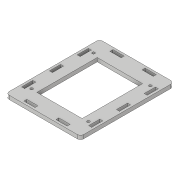
# Autodesk Inventor part: tapa1
Saved by Autodesk Inventor 2019 (Build 230136000, 136)
## iProperties
Created: 2018-09-17
Part Number: tapa1
Material: Genérico
Document SubType Name: Modeling
Designer: lmacia
Density: 1 g/cm^3
Appearance: Valor por defecto
Author: lmacia
Autodesk Inventor part; units mm, degrees
ref_plane "YZ Plane" through (0, 0, 0) normal (1, 0, 0) x (0, 1, 0)
ref_plane "XZ Plane" through (0, 0, 0) normal (0, 1, 0) x (-1, 0, 0)
ref_plane "XY Plane" through (0, 0, 0) normal (0, 0, 1) x (1, 0, 0)
sketch "Boceto1" plane through (0, 0, 0) normal (0, 1, 0) x (-1, 0, 0)
  line L0 (25.8375, 17.5875) -> (25.7625, 17.5875)
  line L1 (25.7625, 17.5875) -> (25.7625, 26.5875)
  line L2 (25.7625, 26.5875) -> (25.8375, 26.5875)
  line L3 (25.7625, 26.5875) -> (28.0125, 26.5875)
  line L4 (28.0875, 26.5875) -> (28.1625, 26.5875)
  line L5 (28.1625, 17.5875) -> (28.0875, 17.5875)
  line L6 (28.0125, 17.5875) -> (25.7625, 17.5875)
  line L7 (25.8148, -4.7625) -> (25.7398, -4.7625)
  line L8 (25.7398, -4.7625) -> (25.7398, 4.2375)
  line L9 (25.7398, 4.2375) -> (25.8148, 4.2375)
  line L10 (25.7398, 4.2375) -> (28.1625, 4.2375)
  line L11 (28.1625, -4.7625) -> (28.0875, -4.7625)
  line L12 (28.0875, -4.7625) -> (25.8148, -4.7625)
  line L13 (23.8875, 23.8875) -> (23.8517, 23.6157)
  line L14 (23.8517, 23.6157) -> (23.7468, 23.3625)
  line L15 (23.754, 23.357) -> (23.5871, 23.1396)
  line L16 (23.58, 23.145) -> (23.3625, 22.9782)
  line L17 (23.3625, 22.9782) -> (23.1093, 22.8733)
  line L18 (23.1093, 22.8733) -> (22.8375, 22.8375)
  line L19 (22.8375, 22.8375) -> (22.5657, 22.8733)
  line L20 (22.5657, 22.8733) -> (22.3125, 22.9782)
  line L21 (22.3125, 22.9782) -> (22.095, 23.145)
  line L22 (22.0879, 23.1396) -> (21.921, 23.357)
  line L23 (21.9282, 23.3625) -> (21.8233, 23.6157)
  line L24 (21.8233, 23.6157) -> (21.7875, 23.8875)
  line L25 (21.7875, 23.8875) -> (21.8233, 24.1593)
  line L26 (21.8233, 24.1593) -> (21.9282, 24.4125)
  line L27 (21.9282, 24.4125) -> (22.095, 24.63)
  line L28 (22.095, 24.63) -> (22.3125, 24.7968)
  line L29 (22.3125, 24.7968) -> (22.5657, 24.9017)
  line L30 (22.5657, 24.9017) -> (22.8375, 24.9375)
  line L31 (22.8387, 24.9464) -> (23.1104, 24.9106)
  line L32 (23.1093, 24.9017) -> (23.3625, 24.7968)
  line L33 (23.3625, 24.7968) -> (23.58, 24.63)
  line L34 (23.58, 24.63) -> (23.7468, 24.4125)
  line L35 (23.7468, 24.4125) -> (23.8517, 24.1593)
  line L36 (23.8517, 24.1593) -> (23.8875, 23.8875)
  line L37 (18.225, 24.3) -> (18.225, -24.3)
  line L38 (18.225, -24.3) -> (-18.225, -24.3)
  line L39 (-18.225, -24.3) -> (-18.225, 24.3)
  line L40 (-18.225, 24.3) -> (18.225, 24.3)
  line L41 (-25.8375, 26.5875) -> (-25.7625, 26.5875)
  line L42 (-25.7625, 26.5875) -> (-25.7625, 17.5875)
  line L43 (-25.7625, 17.5875) -> (-25.8375, 17.5875)
  line L44 (-25.8375, 17.5875) -> (-28.0875, 17.5875)
  line L45 (-28.0875, 17.5875) -> (-28.1625, 17.5875)
  line L46 (-28.1625, 17.5875) -> (-28.1625, 26.5875)
  line L47 (-28.1625, 26.5875) -> (-28.0875, 26.5875)
  line L48 (-28.0875, 26.5875) -> (-25.8375, 26.5875)
  line L49 (-25.8375, -27.1125) -> (-28.0875, -27.1125)
  line L50 (-28.0875, -27.1125) -> (-28.1625, -27.1125)
  line L51 (-28.1625, -27.1125) -> (-28.1625, -18.1125)
  line L52 (-28.1625, -18.1125) -> (-28.0875, -18.1125)
  line L53 (-28.0875, -18.1125) -> (-25.8375, -18.1125)
  line L54 (-25.8375, -18.1125) -> (-25.7625, -18.1125)
  line L55 (-25.7625, -18.1125) -> (-25.7625, -27.1125)
  line L56 (-25.7625, -27.1125) -> (-25.8375, -27.1125)
  line L57 (-22.5657, 22.8733) -> (-22.8375, 22.8375)
  line L58 (-22.8375, 22.8375) -> (-23.1093, 22.8733)
  line L59 (-23.1093, 22.8733) -> (-23.3625, 22.9782)
  line L60 (-23.3625, 22.9782) -> (-23.58, 23.145)
  line L61 (-23.58, 23.145) -> (-23.7468, 23.3625)
  line L62 (-23.7551, 23.3591) -> (-23.86, 23.6123)
  line L63 (-23.8517, 23.6157) -> (-23.8875, 23.8875)
  line L64 (-23.8875, 23.8875) -> (-23.8517, 24.1593)
  line L65 (-23.8517, 24.1593) -> (-23.7468, 24.4125)
  line L66 (-23.7468, 24.4125) -> (-23.58, 24.63)
  line L67 (-23.58, 24.63) -> (-23.3625, 24.7968)
  line L68 (-23.3625, 24.7968) -> (-23.1093, 24.9017)
  line L69 (-23.1093, 24.9017) -> (-22.8375, 24.9375)
  line L70 (-22.8363, 24.9464) -> (-22.5646, 24.9106)
  line L71 (-22.5657, 24.9017) -> (-22.3125, 24.7968)
  line L72 (-22.3125, 24.7968) -> (-22.095, 24.63)
  line L73 (-22.095, 24.63) -> (-21.9282, 24.4125)
  line L74 (-21.9282, 24.4125) -> (-21.8233, 24.1593)
  line L75 (-21.8233, 24.1593) -> (-21.7875, 23.8875)
  line L76 (-21.7875, 23.8875) -> (-21.8233, 23.6157)
  line L77 (-21.8233, 23.6157) -> (-21.9282, 23.3625)
  line L78 (-21.9282, 23.3625) -> (-22.095, 23.145)
  line L79 (-22.095, 23.145) -> (-22.3125, 22.9782)
  line L80 (-22.3091, 22.9699) -> (-22.5623, 22.865)
  line L81 (-28.1625, -4.7625) -> (-28.1625, 4.2375)
  line L82 (-28.1625, 4.2375) -> (-28.0875, 4.2375)
  line L83 (-28.0875, 4.2375) -> (-25.8375, 4.2375)
  line L84 (-25.8375, 4.2375) -> (-25.7625, 4.2375)
  line L85 (-25.7625, 4.2375) -> (-25.7625, -4.7625)
  line L86 (-25.7625, -4.7625) -> (-25.8375, -4.7625)
  line L87 (-25.8375, -4.7625) -> (-28.0875, -4.7625)
  line L88 (-28.0875, -4.7625) -> (-28.1625, -4.7625)
  line L89 (-22.5657, -27.0017) -> (-22.8375, -27.0375)
  line L90 (-22.8375, -27.0375) -> (-23.1093, -27.0017)
  line L91 (-23.1093, -27.0017) -> (-23.3625, -26.8968)
  line L92 (-23.3625, -26.8968) -> (-23.58, -26.73)
  line L93 (-23.58, -26.73) -> (-23.7468, -26.5125)
  line L94 (-23.7551, -26.5159) -> (-23.86, -26.2627)
  line L95 (-23.8517, -26.2593) -> (-23.8875, -25.9875)
  line L96 (-23.8875, -25.9875) -> (-23.8517, -25.7157)
  line L97 (-23.8517, -25.7157) -> (-23.7468, -25.4625)
  line L98 (-23.7468, -25.4625) -> (-23.58, -25.245)
  line L99 (-23.58, -25.245) -> (-23.3625, -25.0782)
  line L100 (-23.3625, -25.0782) -> (-23.1093, -24.9733)
  line L101 (-23.1093, -24.9733) -> (-22.8375, -24.9375)
  line L102 (-22.8363, -24.9286) -> (-22.5646, -24.9644)
  line L103 (-22.5657, -24.9733) -> (-22.3125, -25.0782)
  line L104 (-22.3125, -25.0782) -> (-22.095, -25.245)
  line L105 (-22.095, -25.245) -> (-21.9282, -25.4625)
  line L106 (-21.9282, -25.4625) -> (-21.8233, -25.7157)
  line L107 (-21.8233, -25.7157) -> (-21.7875, -25.9875)
  line L108 (-21.7875, -25.9875) -> (-21.8233, -26.2593)
  line L109 (-21.8233, -26.2593) -> (-21.9282, -26.5125)
  line L110 (-21.9282, -26.5125) -> (-22.095, -26.73)
  line L111 (-22.0896, -26.7371) -> (-22.307, -26.904)
  line L112 (-22.3125, -26.8968) -> (-22.5657, -27.0017)
  line L113 (8.4187, -36.0375) -> (8.4187, -33.7875)
  line L114 (8.4187, -33.7875) -> (8.4187, -33.7125)
  line L115 (8.4187, -33.7125) -> (17.4187, -33.7125)
  line L116 (17.4187, -33.7125) -> (17.4187, -33.7875)
  line L117 (17.4187, -33.7875) -> (17.4187, -36.0375)
  line L118 (17.4187, -36.0375) -> (17.4187, -36.1125)
  line L119 (17.4187, -36.1125) -> (8.4187, -36.1125)
  line L120 (8.4187, -36.1125) -> (8.4187, -36.0375)
  line L121 (8.4187, 33.1875) -> (8.4187, 33.2625)
  line L122 (8.4187, 33.1875) -> (8.4187, 35.5125)
  line L123 (8.4187, 35.5125) -> (8.4187, 35.5875)
  line L124 (17.4187, 35.5875) -> (17.4187, 35.5125)
  line L125 (17.4187, 33.1875) -> (8.4187, 33.1875)
  line L126 (-17.4188, 33.1875) -> (-17.4188, 33.2625)
  line L127 (-17.4188, 33.2625) -> (-17.4188, 35.5125)
  line L128 (-17.4188, 35.5125) -> (-17.4188, 35.5875)
  line L129 (-17.4188, 35.5875) -> (-8.4188, 35.5875)
  line L130 (-8.4188, 35.5875) -> (-8.4188, 35.5125)
  line L131 (-8.4188, 35.5125) -> (-8.4188, 33.2625)
  line L132 (-8.4188, 33.2625) -> (-8.4188, 33.1875)
  line L133 (-8.4188, 33.1875) -> (-17.4188, 33.1875)
  line L134 (-8.4188, -33.7125) -> (-8.4188, -33.7875)
  line L135 (-8.4188, -33.7875) -> (-8.4188, -36.0375)
  line L136 (-8.4188, -36.0375) -> (-8.4188, -36.1125)
  line L137 (-8.4188, -36.1125) -> (-17.4188, -36.1125)
  line L138 (-17.4188, -36.1125) -> (-17.4188, -36.0375)
  line L139 (-17.4188, -36.0375) -> (-17.4188, -33.7875)
  line L140 (-17.4188, -33.7875) -> (-17.4188, -33.7125)
  line L141 (-17.4188, -33.7125) -> (-8.4188, -33.7125)
  line L142 (23.8517, -25.7157) -> (23.8875, -25.9875)
  line L143 (23.8875, -25.9875) -> (23.8517, -26.2593)
  line L144 (23.8517, -26.2593) -> (23.7468, -26.5125)
  line L145 (23.7468, -26.5125) -> (23.58, -26.73)
  line L146 (23.5854, -26.7371) -> (23.368, -26.904)
  line L147 (23.3625, -26.8968) -> (23.1093, -27.0017)
  line L148 (23.1093, -27.0017) -> (22.8375, -27.0375)
  line L149 (22.8375, -27.0375) -> (22.5657, -27.0017)
  line L150 (22.5657, -27.0017) -> (22.3125, -26.8968)
  line L151 (22.3125, -26.8968) -> (22.095, -26.73)
  line L152 (22.095, -26.73) -> (21.9282, -26.5125)
  line L153 (21.9282, -26.5125) -> (21.8233, -26.2593)
  line L154 (21.8233, -26.2593) -> (21.7875, -25.9875)
  line L155 (21.7875, -25.9875) -> (21.8233, -25.7157)
  line L156 (21.8233, -25.7157) -> (21.9282, -25.4625)
  line L157 (21.9282, -25.4625) -> (22.095, -25.245)
  line L158 (22.0896, -25.2379) -> (22.307, -25.071)
  line L159 (22.3125, -25.0782) -> (22.5657, -24.9733)
  line L160 (22.5657, -24.9733) -> (22.8375, -24.9375)
  line L161 (22.8375, -24.9375) -> (23.1093, -24.9733)
  line L162 (23.1093, -24.9733) -> (23.3625, -25.0782)
  line L163 (23.368, -25.071) -> (23.5854, -25.2379)
  line L164 (23.58, -25.245) -> (23.7468, -25.4625)
  line L165 (23.7468, -25.4625) -> (23.8517, -25.7157)
  line L166 (25.7625, -27.1125) -> (25.7625, -18.1125)
  line L167 (25.7625, -18.1125) -> (25.8375, -18.1125)
  line L168 (25.8375, -18.1125) -> (28.0875, -18.1125)
  line L169 (28.0875, -18.1125) -> (28.1625, -18.1125)
  line L170 (28.1625, -18.1125) -> (28.1625, -27.1125)
  line L171 (28.1625, -27.1125) -> (28.0875, -27.1125)
  line L172 (28.0875, -27.1125) -> (25.8375, -27.1125)
  line L173 (25.8375, -27.1125) -> (25.7625, -27.1125)
  line L174 (29.9643, -35.2893) -> (29.9643, 34.7644)
  line L175 (27.3393, 37.3894) -> (-27.3449, 37.3893)
  line L176 (-29.9643, 34.7886) -> (-29.9643, -35.2893)
  line L177 (-27.3391, -37.9143) -> (27.3393, -37.9143)
  arc A0 (-27.3449, 37.3893) -> (-29.9643, 34.7886) centre (-27.3636, 34.7886) ccw
  arc A1 (27.3393, -37.9143) -> (29.9643, -35.2893) centre (27.3393, -35.2893) ccw
  arc A2 (29.9643, 34.7644) -> (27.3393, 37.3894) centre (27.3394, 34.7644) ccw
  arc A3 (-29.9643, -35.2893) -> (-27.3391, -37.9143) centre (-26.3784, -34.3283) ccw
  line L178 (17.4187, -36.1125) -> (8.4187, -36.1125)
  line L179 (8.4187, -36.1125) -> (8.4187, -33.7125)
  line L180 (8.4187, -33.7125) -> (17.4187, -33.7125)
  line L181 (17.4187, -33.7125) -> (17.4187, -36.1125)
  line L182 (-8.4188, -36.1125) -> (-17.4188, -36.1125)
  line L183 (-17.4188, -36.1125) -> (-17.4188, -33.7125)
  line L184 (-17.4188, -33.7125) -> (-8.4188, -33.7125)
  line L185 (-8.4188, -33.7125) -> (-8.4188, -36.1125)
  line L186 (-25.7625, -27.1125) -> (-28.1625, -27.1125)
  line L187 (-28.1625, -27.1125) -> (-28.1625, -18.1125)
  line L188 (-28.1625, -18.1125) -> (-25.7625, -18.1125)
  line L189 (-25.7625, -18.1125) -> (-25.7625, -27.1125)
  line L190 (-25.7625, -4.7625) -> (-28.1625, -4.7625)
  line L191 (-28.1625, -4.7625) -> (-28.1625, 4.2375)
  line L192 (-28.1625, 4.2375) -> (-25.7625, 4.2375)
  line L193 (-25.7625, 4.2375) -> (-25.7625, -4.7625)
  line L194 (-25.7625, 17.5875) -> (-28.1625, 17.5875)
  line L195 (-28.1625, 17.5875) -> (-28.1625, 26.5875)
  line L196 (-28.1625, 26.5875) -> (-25.7625, 26.5875)
  line L197 (-25.7625, 26.5875) -> (-25.7625, 17.5875)
  line L198 (-17.4188, 33.1875) -> (-8.4188, 33.1875)
  line L199 (-8.4188, 33.1875) -> (-8.4188, 35.5875)
  line L200 (-8.4188, 35.5875) -> (-17.4188, 35.5875)
  line L201 (-17.4188, 35.5875) -> (-17.4188, 33.1875)
  line L202 (8.4187, 33.1875) -> (17.4187, 33.1875)
  line L203 (17.4187, 33.1875) -> (17.4187, 35.5875)
  line L204 (17.4187, 35.5875) -> (8.4187, 35.5875)
  line L205 (8.4187, 35.5875) -> (8.4187, 33.1875)
  line L206 (25.7625, 26.5875) -> (28.1625, 26.5875)
  line L207 (28.1625, 26.5875) -> (28.1625, 17.5875)
  line L208 (28.1625, 17.5875) -> (25.7625, 17.5875)
  line L209 (25.7625, 17.5875) -> (25.7625, 26.5875)
  line L210 (25.7398, 4.2375) -> (28.1398, 4.2375)
  line L211 (28.1398, 4.2375) -> (28.1398, -4.7625)
  line L212 (28.1398, -4.7625) -> (25.7398, -4.7625)
  line L213 (25.7398, -4.7625) -> (25.7398, 4.2375)
  line L214 (28.1625, -27.1125) -> (25.7625, -27.1125)
  line L215 (25.7625, -27.1125) -> (25.7625, -18.1125)
  line L216 (25.7625, -18.1125) -> (28.1625, -18.1125)
  line L217 (28.1625, -18.1125) -> (28.1625, -27.1125)
  circle A4 centre (22.8375, 23.8875) radius 1.05
  circle A5 centre (22.8375, -25.9875) radius 1.05
  circle A6 centre (-22.8375, -25.9875) radius 1.05
  circle A7 centre (-22.8375, 23.8875) radius 1.05
  point P0 (0, 0)
  dimension "d1" = 2.4
  dimension "d2" = 9
  dimension "d5" = 2.1
  dimension "d6" = 2.1
  dimension "d7" = 2.1
  dimension "d8" = 2.1
  constraints: 436 end point, 20 parallel, 12 tangent, 11 horizontal, 10 perpendicular, 8 centre point, 8 point on circle
  measures "d1" distance of L211.end L212.end
  measures "d2" distance of L210.end L211.end
  measures "d5" diameter of A4
  measures "d6" diameter of A7
  measures "d7" diameter of A6
  measures "d8" diameter of A5
extrude "Extrusión1" add sketch "Boceto1" along normal blind 3
